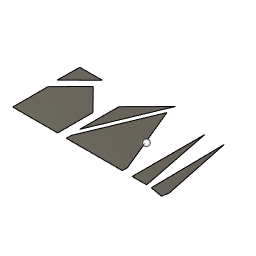
Paper_Meshes (Autodesk Fusion 360 design; units mm, degrees)
Autodesk Fusion 360 part; units mm, degrees
sketch "Sketch3" plane through (0, 0, 0) normal (0, 0, 1) x (1, 0, 0)
  line L0 (0, 20) -> (0, 21)
  line L1 (0, 21) -> (0.859812, 20.48939)
  line L2 (0, 20) -> (0.869083, 20.494667)
  dimension "d3" = 1
  dimension "d4" = 1
  dimension "d5" = 1
  constraint vertical L0
  measures "d3" distance of L0.start L0.end
sketch "Sketch4" plane through (-8.598125, 15.106099, 0) normal (0.494667, -0.869083, 0) x (0.869083, 0.494667, 0)
  line L0 (9.893332, 0) -> (10.882665, 0)
  line L1 (10.882665, 0) -> (10.882665, 0.25)
  line L2 (10.882665, 0.25) -> (9.893332, 0.25)
  line L3 (9.893332, 0.25) -> (9.893332, 0)
sketch "Sketch9" plane through (0, 0, 0) normal (0, 0, 1) x (1, 0, 0)
sketch "Sketch8" plane through (0, 0, 0) normal (0, 0, 1) x (1, 0, 0)
sketch "Sketch6" plane through (0, 0, 0) normal (0, 0, 1) x (1, 0, 0)
  line L0 (0.5, 0.6) -> (0.926, 0.6)
  line L1 (0.926, 0.6) -> (0.494335, 0.176101)
  line L2 (0.494335, 0.176101) -> (0.5, 0.6)
  line L3 (1.3, 0.6) -> (2.15, 0.6)
  line L4 (2.15, 0.6) -> (2.15, -0.5)
  line L5 (2.15, -0.5) -> (1.3, -0.5)
  line L6 (1.3, -0.5) -> (1.3, 0.6)
  line L7 (1.725, 0.6) -> (1.293335, 0.176101)
  line L8 (1.725, 0.6) -> (2.148899, 0.168335)
  dimension "d16" = 0.426
  dimension "d17" = 0.605
  dimension "d18" = 0.85
  dimension "d19" = 1.1
  dimension "d20" = 0.605
  dimension "d21" = 0.605
  constraint horizontal L0
  constraint horizontal L3
  constraint vertical L4
  constraint horizontal L5
  constraint vertical L6
  constraint midpoint L3 L7.start
  constraint parallel L1 L7
  constraint perpendicular L7 L8
  measures "d16" distance of L0.start L0.end
  measures "d18" distance of L3.start L3.end
  measures "d19" distance of L3.start L5.end
extrude "Extrude4" add sketch "Sketch6" along normal blind 1 contours L0 L1 L2 picked at (0.640112, 0.4587) makes body 1
sketch "Sketch7" plane through (0, 0, 0) normal (0, 0, 1) x (1, 0, 0)
  line L0 (1.2, 0.6) -> (2.05, 0.6)
  line L1 (2.05, 0.6) -> (2.05, -0.5)
  line L2 (2.05, -0.5) -> (1.2, -0.5)
  line L3 (1.2, -0.5) -> (1.2, 0.6)
  line L4 (1.625, 0.6) -> (1.2, 0.169419)
  line L5 (1.625, 0.6) -> (1.625, -0.005)
  line L6 (1.625, -0.005) -> (1.2, -0.424107)
  line L7 (1.625, -0.005) -> (2.221888, -0.005) construction
  line L8 (1.2, -0.424107) -> (1.625, 0.6)
  line L9 (1.625, 0.6) -> (2.05, -0.424107)
  dimension "d24" = 0.85
  dimension "d25" = 1.1
  dimension "d26" = 0.605
  dimension "d27" = 0.605
  dimension "d28" = 135.4
  constraint horizontal L0
  constraint perpendicular L0 L1
  constraint perpendicular L1 L2
  constraint perpendicular L0 L3
  constraint midpoint L0 L4.start
  constraint perpendicular L0 L5
  constraint horizontal L7
  measures "d24" distance of L0.start L0.end
  measures "d25" distance of L0.end L1.end
  measures "d27" distance of L4.start L5.end
  measures "d28" angle of L6 L7
extrude "Extrude5" add sketch "Sketch7" along normal blind 0.1 separate body contours L3 L4 L8 picked at (1.341667, 0.115104) makes body 2
extrude "Extrude6" cut 1 faces at (0.640112, 0.4587, 1) along direction (0, 0, -1) blind 0.9 on bodies 1 bodies 1
sketch "Sketch10" plane through (0, 0, 0) normal (0, 0, 1) x (1, 0, 0)
  line L0 (-0.8, 0.7) -> (0.05, 0.7)
  line L1 (0.05, 0.7) -> (0.05, -0.4)
  line L2 (0.05, -0.4) -> (-0.8, -0.4)
  line L3 (-0.8, 0.7) -> (-0.8, -0.4)
  line L4 (-0.375, 0.7) -> (-0.8, 0.269419)
  line L5 (-0.375, 0.7) -> (0.05, 0.269419)
  dimension "d33" = 0.85
  dimension "d34" = 1.1
  dimension "d35" = 0.85
  dimension "d36" = 0.605
  dimension "d37" = 0.605
  constraint horizontal L0
  constraint perpendicular L0 L1
  constraint perpendicular L1 L2
  constraint midpoint L0 L4.start
  measures "d33" distance of L0.start L0.end
  measures "d34" distance of L0.end L1.end
  measures "d35" distance of L1.end L2.end
extrude "Extrude7" add sketch "Sketch10" along normal blind 0.1 separate body contours L1 L2 L3 L4 L5 picked at (-0.516667, 0.046279) makes body 3
sketch "Sketch11" plane through (0, 0, 0) normal (0, 0, 1) x (1, 0, 0)
  line L0 (2, 0.6) -> (2.85, 0.6)
  line L1 (2.85, 0.6) -> (2.85, -0.5)
  line L2 (2.85, -0.5) -> (2, -0.5)
  line L3 (2, -0.5) -> (2, 0.6)
  line L4 (2.425, 0.6) -> (2, 0.169419)
  line L5 (2.425, 0.6) -> (2.85, 0.169419)
  line L6 (2.425, -0.005) -> (3.021888, -0.005) construction
  line L7 (2, -0.424107) -> (2.425, 0.6)
  line L8 (2.425, 0.6) -> (2.85, -0.424107)
  dimension "d40" = 0.85
  dimension "d41" = 1.1
  dimension "d42" = 0.605
  dimension "d43" = 0.605
  dimension "d44" = 0.605
  constraint horizontal L0
  constraint vertical L1
  constraint horizontal L2
  constraint vertical L3
  constraint midpoint L0 L4.start
  constraint horizontal L6
  measures "d40" distance of L0.start L0.end
  measures "d41" distance of L0.start L2.end
  measures "d44" distance of L4.start L6.start
extrude "Extrude8" add sketch "Sketch11" along normal blind 0.1 separate body contours L1 L2 L3 L7 L8 picked at (2.425, -0.082738) makes body 4
sketch "Sketch12" plane through (0, 0, 0) normal (0, 0, 1) x (1, 0, 0)
  line L0 (-1.9, 0.7) -> (-1.05, 0.7)
  line L1 (-1.05, 0.7) -> (-1.05, -0.4)
  line L2 (-1.05, -0.4) -> (-1.9, -0.4)
  line L3 (-1.9, -0.4) -> (-1.9, 0.7)
  line L4 (-1.475, 0.7) -> (-1.475, -0.4)
  line L5 (-1.9, -0.335976) -> (-1.475, 0.7)
  line L6 (-1.475, 0.7) -> (-1.05, -0.335976)
  line L7 (-1.2625, -0.367988) -> (-1.475, 0.7)
  line L8 (-1.2625, -0.367988) -> (-1.25613, -0.4)
  line L9 (-1.9, -0.335976) -> (-1.475, -0.4)
  line L10 (-1.475, 0.7) -> (-1.7, -0.4)
  dimension "d48" = 0.85
  dimension "d49" = 1.1
  constraint horizontal L0
  constraint vertical L1
  constraint horizontal L2
  constraint vertical L3
  constraint midpoint L0 L4.start
  constraint perpendicular L0 L4
  constraint coincident L2 L4.end
  constraint parallel L7 L8
  constraint coincident L2 L10.end
  measures "d48" distance of L0.start L0.end
  measures "d49" distance of L0.start L2.end
extrude "Extrude9" add sketch "Sketch12" along normal blind 0.1 separate body contours L2 L4 L7 L8 picked at (-1.404167, -0.022663) makes body 5
sketch "Sketch13" plane through (0, 0, 0) normal (0, 0, 1) x (1, 0, 0)
  line L0 (-1.7, 0.7) -> (-2.55, 0.7)
  line L1 (-2.55, 0.7) -> (-2.55, -0.4)
  line L2 (-2.55, -0.4) -> (-1.7, -0.4)
  line L3 (-1.7, -0.4) -> (-1.7, 0.7)
  line L4 (-2.1, 0.7) -> (-1.7, 0.2461)
  line L5 (-2.1, 0.7) -> (-2.1, -0.4)
  line L6 (-2.55, 0.095) -> (-2.661777, 0.095) construction
  line L7 (-1.7, -0.299454) -> (-2.1, 0.7)
  line L8 (-1.890422, -0.4) -> (-2.1, 0.7)
  dimension "d55" = 0.85
  dimension "d56" = 1.1
  dimension "d57" = 0.605
  constraint horizontal L0
  constraint vertical L1
  constraint horizontal L2
  constraint vertical L3
  constraint coincident L0 L4.start
  constraint coincident L3 L4.end
  constraint perpendicular L0 L5
  constraint horizontal L6
  constraint coincident L2 L5.end
  constraint coincident L1 L6.start
  measures "d55" distance of L0.start L0.end
  measures "d56" distance of L0.start L2.end
  measures "d57" distance of L4.start L4.end
extrude "Extrude10" add sketch "Sketch13" along normal blind 0.1 separate body contours L2 L3 L7 L8 picked at (-1.896807, 0.000182) makes body 6
move_body "Move1" bodies 6 to x (0.98480775, -0.17364818, 0) y (0.17364818, 0.98480775, 0) z (0, 0, 1) at (0.037556, -0.370738, 0)
sketch "Sketch14" plane through (0, 0, 0) normal (0, 0, 1) x (1, 0, 0)
scale "Scale1" factors (2000, 2000, 2) about (0.494335, 0.176101, 0.1) bodies 1
scale "Scale2" factors (2000, 2000, 2) about (0.05, 0.269419, 0.1) bodies 3
scale "Scale3" factors (2500, 2500, 2) about (2.425, 0.6, 0.1) bodies 4
scale "Scale4" factors (2500, 2500, 2) about (1.2, -0.424107, 0) bodies 2
scale "Scale5" factors (2500, 2500, 5) about (-1.25613, -0.4, 0.1) bodies 5
scale "Scale6" factors (2500, 2500, 4) about (-1.688617, -0.37044, 0.1) bodies 6
move_body "Move2" bodies 3 to x (1, 0, 0) y (0, 1, 0) z (0, 0, 1) at (-2000, 0, 0)
move_body "Move3" bodies 1 to x (1, 0, 0) y (0, 1, 0) z (0, 0, 1) at (-3744.302517, 387.55472, 0)
move_body "Move4" bodies 4 to x (1, 0, 0) y (0, 1, 0) z (0, 0, 1) at (-400, 1400, 0)
move_body "Move5" bodies 2 to x (1, 0, 0) y (0, 1, 0) z (0, 0, 1) at (-1500, -800, 0)
move_body "Move6" bodies 5 to x (1, 0, 0) y (0, 1, 0) z (0, 0, 1) at (1802.91069, -1374.595593, 0)
move_body "Move7" bodies 5 to x (1, 0, 0) y (0, 1, 0) z (0, 0, 1) at (-411.824299, 20.018666, 0)
move_body "Move8" bodies 4 to x (1, 0, 0) y (0, 1, 0) z (0, 0, 1) at (-200, 0, 0)
move_body "Move9" bodies 2 to x (1, 0, 0) y (0, 1, 0) z (0, 0, 1) at (-200, 0, 0)
move_body "Move10" bodies 6 to x (1, 0, 0) y (0, 1, 0) z (0, 0, 1) at (2089.410256, -1197.64969, 0)
named bodies: "Puzzle2_Mesh_Folds", "Puzzle3_Mesh_Folds", "Puzzles2_Mesh_Body", "Puzzle3_Mesh_Body", "Puzzle4_Mesh_Body", "Puzzle4_Mesh_Folds"
